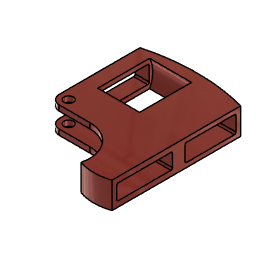
Outer Cage (Autodesk Fusion 360 design; units mm, degrees)
Autodesk Fusion 360 part; units mm, degrees
sketch "Sketch2" plane through (0, 0, 0) normal (0, 0, 1) x (1, 0, 0)
  line L0 (0, 104.0152) -> (0, 0)
  arc A0 (0, 0) -> (11.3958, -11.9848) centre (12, 0) ccw
  line L1 (11.3958, -11.9848) -> (51.3958, -11.9848)
  arc A1 (130, 104.0152) -> (0, 104.0152) centre (65, -137.3869) ccw
  line L2 (130, 104.0152) -> (130, -61.9848)
  arc A2 (90, -61.9848) -> (130, -61.9848) centre (110, -5.4163) ccw
  arc A3 (90, -61.9848) -> (51.3958, -11.9848) centre (51.2702, -51.9846) ccw
  dimension "d1" = 166
  dimension "d2" = 12
  dimension "d3" = 40
  dimension "d4" = 116
  dimension "d5" = 40
  dimension "d6" = 60
  dimension "d7" = 40
  dimension "d8" = 130
  dimension "d9" = 250
  constraint coincident L0.end A0.start
  constraint horizontal L1
  constraint vertical L2
  constraint vertical L0
  constraint horizontal L0.start A1.start
  constraint horizontal L2.end A2.start
  constraint tangent L0 A0
  measures "d1" distance of A1.start L2.end
  measures "d2" radius of A0
  measures "d3" distance of A0.end L1.end
  measures "d4" distance of L0.start L1
  measures "d5" radius of A3
  measures "d6" radius of A2
  measures "d7" horizontal distance of L2.end A2.start
  measures "d8" distance of L0 L2
  measures "d9" radius of A1
extrude "Extrude1" add sketch "Sketch2" along normal mid plane 34
sketch "Sketch3" plane through (130, 0, 0) normal (1, 0, 0) x (0, 1, 0)
  line L0 (104.0152, -17) -> (104.0152, 17)
  line L1 (104.0152, 17) -> (-61.9848, 17)
  line L2 (-61.9848, 17) -> (-61.9848, -17)
  line L3 (-61.9848, -17) -> (104.0152, -17)
  line L4 (-53.9848, 10) -> (14.0152, 10)
  line L5 (16.0152, 8) -> (16.0152, -8)
  line L6 (14.0152, -10) -> (-53.9848, -10)
  line L7 (-55.9848, -8) -> (-55.9848, 8)
  line L8 (-55.9848, 10) -> (16.0152, -10) construction
  line L9 (16.0152, 10) -> (-55.9848, -10) construction
  line L10 (34.0152, 11.25) -> (96.0152, 11.25)
  line L11 (98.0152, 9.25) -> (98.0152, -9.25)
  line L12 (96.0152, -11.25) -> (34.0152, -11.25)
  line L13 (32.0152, -9.25) -> (32.0152, 9.25)
  line L14 (32.0152, 11.25) -> (98.0152, -11.25) construction
  line L15 (98.0152, 11.25) -> (32.0152, -11.25) construction
  arc A0 (-53.9848, 10) -> (-55.9848, 8) centre (-53.9848, 8) ccw
  arc A1 (-55.9848, -8) -> (-53.9848, -10) centre (-53.9848, -8) ccw
  arc A2 (14.0152, -10) -> (16.0152, -8) centre (14.0152, -8) ccw
  arc A3 (16.0152, 8) -> (14.0152, 10) centre (14.0152, 8) ccw
  arc A4 (34.0152, 11.25) -> (32.0152, 9.25) centre (34.0152, 9.25) ccw
  arc A5 (98.0152, 9.25) -> (96.0152, 11.25) centre (96.0152, 9.25) ccw
  arc A6 (96.0152, -11.25) -> (98.0152, -9.25) centre (96.0152, -9.25) ccw
  arc A7 (32.0152, -9.25) -> (34.0152, -11.25) centre (34.0152, -9.25) ccw
  point P0 (-19.9848, 0)
  point P1 (65.0152, 0)
  dimension "d12" = 72
  dimension "d13" = 66
  dimension "d14" = 22.5
  dimension "d15" = 20
  dimension "d16" = 6
  dimension "d17" = 6
  dimension "d18" = 2
  dimension "d19" = 2
  dimension "d20" = 2
  dimension "d21" = 2
  dimension "d22" = 2
  dimension "d23" = 2
  dimension "d24" = 2
  dimension "d25" = 2
  constraint horizontal L4
  constraint perpendicular L4 L5
  constraint parallel L4 L6
  constraint parallel L5 L7
  constraint coincident L8 P0
  constraint coincident L9 P0
  constraint horizontal L10
  constraint perpendicular L10 L11
  constraint parallel L10 L12
  constraint parallel L11 L13
  constraint coincident L14 P1
  constraint coincident L15 P1
  constraint horizontal origin P1
  constraint horizontal P0 P1
  constraint coincident L8.start L7
  constraint coincident L8.start L4
  constraint tangent L7 A0
  constraint tangent L4 A0
  constraint coincident L9.end L7
  constraint coincident L9.end L6
  constraint tangent L7 A1
  constraint tangent L6 A1
  constraint coincident L8.end L6
  constraint coincident L8.end L5
  constraint tangent L6 A2
  constraint tangent L5 A2
  constraint coincident L9.start L4
  constraint coincident L9.start L5
  constraint tangent L4 A3
  constraint tangent L5 A3
  constraint coincident L14.start L13
  constraint coincident L14.start L10
  constraint tangent L13 A4
  constraint tangent L10 A4
  constraint coincident L15.start L10
  constraint coincident L15.start L11
  constraint tangent L10 A5
  constraint tangent L11 A5
  constraint coincident L14.end L11
  constraint coincident L14.end L12
  constraint tangent L11 A6
  constraint tangent L12 A6
  constraint coincident L15.end L13
  constraint coincident L15.end L12
  constraint tangent L13 A7
  constraint tangent L12 A7
  measures "d12" distance of L8.start L9.start
  measures "d13" distance of L14.start L15.start
  measures "d14" distance of L15.start L14.end
  measures "d15" distance of L8.start L9.end
  measures "d16" distance of L2 L7
  measures "d17" distance of L0 L11
  measures "d18" radius of A0
  measures "d19" radius of A1
  measures "d20" radius of A2
  measures "d21" radius of A3
  measures "d22" radius of A4
  measures "d23" radius of A5
  measures "d24" radius of A6
  measures "d25" radius of A7
extrude "Extrude2" cut sketch "Sketch3" against normal through all contours L4 L5 L6 L7 A0 A1 A2 A3 | L10 L11 L12 L13 A4 A5 A6 A7
ref_plane "WorkPlane1" through (45, 21.0152, 0) normal (1, 0, 0) x (0, 1, 0)
sketch "Sketch4" plane through (45, 0, 0) normal (1, 0, 0) x (0, 1, 0)
  circle A0 centre (65.0152, 0) radius 37.5
  line L0 (32.0152, -9.25) -> (32.0152, 9.25)
  dimension "d28" = 75
  dimension "d29" = 33
  constraint horizontal origin A0.centre
  measures "d28" diameter of A0
  measures "d29" distance of A0.centre L0
extrude "Extrude3" cut sketch "Sketch4" along normal mid plane 54
sketch "Sketch5" plane through (0, 0, 17) normal (0, 0, 1) x (-1, 0, 0)
  line L0 (-18, -31.5899) -> (-18, -98.4405)
  line L1 (-18, -98.4405) -> (-72, -98.4405)
  line L2 (-72, -98.4405) -> (-72, -31.5899)
  line L3 (-72, -31.5899) -> (-18, -31.5899)
  arc A0 (-130, -104.0152) -> (0, -104.0152) centre (-65, 137.3869) ccw
  line L4 (0, -104.0152) -> (0, 0)
  arc A1 (0, 0) -> (-11.3958, 11.9848) centre (-12, 0) ccw
  line L5 (-11.3958, 11.9848) -> (-51.3958, 11.9848)
  arc A2 (-90, 61.9848) -> (-51.3958, 11.9848) centre (-51.2702, 51.9846) ccw
  arc A3 (-90, 61.9848) -> (-130, 61.9848) centre (-110, 5.4163) ccw
  line L6 (-130, 61.9848) -> (-130, -104.0152)
  circle A4 centre (-12, 0) radius 6
  dimension "d32" = 12
  constraint concentric A1 A4
  measures "d32" diameter of A4
extrude "Extrude4" cut sketch "Sketch5" against normal blind 34 contours A4
